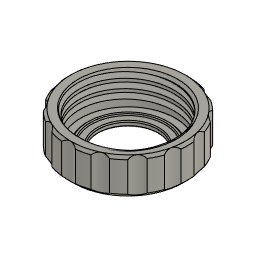
EnfamilTravelBottleNippleAdapter v7 (Autodesk Fusion 360 design; units mm, degrees)
Autodesk Fusion 360 part; units mm, degrees
sketch "Sketch1" plane through (0, 0, 0) normal (0, 1, 0) x (1, 0, 0)
  line L0 (0, 0) -> (0, -15) construction
  line L1 (12, 0) -> (12, -2)
  line L2 (14.7, -2) -> (14.7, -2.4)
  line L3 (14.7, -2.4) -> (16.3, -2.4)
  line L4 (16.3, -2.4) -> (16.3, -2)
  line L5 (16.3, -2) -> (19, -2)
  line L6 (19, -2) -> (19, -15)
  line L7 (19, -15) -> (24, -15)
  line L8 (24, -15) -> (24, 0)
  line L9 (24, 0) -> (12, 0)
  line L10 (12, -2) -> (14.7, -2)
  line L11 (0, -15) -> (0.379, -15)
  line L12 (0.379, -15) -> (19, -15) construction
  line L13 (0, 0) -> (12, 0) construction
  dimension "d1" = 15
  dimension "d2" = 12
  dimension "d3" = 19
  dimension "d4" = 1.6
  dimension "d5" = 0.4
  dimension "d6" = 2
  dimension "d7" = 5
  constraint coincident L0.start L13.start
  constraint vertical L0
  constraint parallel L0 L1
  constraint perpendicular L1 L3
  constraint perpendicular L3 L4
  constraint perpendicular L4 L5
  constraint perpendicular L3 L6
  constraint perpendicular L6 L7
  constraint perpendicular L7 L8
  constraint perpendicular L1 L9
  constraint perpendicular L2 L10
  constraint collinear L5 L10
  constraint equal L5 L10
  constraint perpendicular L0 L11
  constraint perpendicular L0 L12
  constraint perpendicular L1 L13
  measures "d1" distance of L0.start L0.end
  measures "d2" distance of L0 L1
  measures "d3" distance of L0 L6
  measures "d4" distance of L2.end L3.end
  measures "d5" distance of L2.start L2.end
  measures "d6" distance of L1.start L1.end
  measures "d7" distance of L6.end L7.end
revolve "Revolve1" add sketch "Sketch1" angle 360 about axis through (0, 0, 0) along (0, 0, 1)
ref_plane "WorkPlane1" through (0, 0, 4.5) normal (0, 0, 1) x (1, 0, 0)
chamfer "Chamfer1" distance 2 angle 45 1 edges at (-22.3759, -8.6788, 0)
chamfer "Chamfer1" distance 1 angle 45 1 edges at (-22.3759, -8.6788, 15)
chamfer "Chamfer1" distance 1 angle 45 1 edges at (-17.7142, -6.8707, 15)
chamfer "Chamfer1" distance 0.4 angle 45 2 edges at (-11.1879, -4.3394, 2) (-11.1879, -4.3394, 0)
chamfer "Chamfer1" distance 0.4 angle 45 2 edges at (-15.1969, -5.8943, 2.4) (-13.7052, -5.3157, 2.4)
sketch "Sketch5" plane through (0, 0, 15) normal (0, 0, 1) x (-1, 0, 0)
  circle A0 centre (0, 0) radius 23
  circle A1 centre (0, 0) radius 20
  circle A2 centre (0, 28) radius 5
  dimension "d22" = 10
  dimension "d23" = 28
  measures "d22" diameter of A2
  measures "d23" distance of A0.centre A2.centre
extrude "Extrude1" cut sketch "Sketch5" against normal through all contours A2
pattern_circular "C-Pattern1" count 14 over 360 about axis through (0, 0, 1.75) along (0, 0, 1) of "Extrude1"
coil "CoilPrimitive1" cut diameter 38 section triangle out size 2 outside turns 3.5 pitch 3.6 right hand placed x (1, 0, 0) y (0, 1, 0) z (0, 0, 1) at (0, 0, 4.5)
equation "d3 = ( 38 / 2 ) * 1 mm"
named bodies: "TravelBottleNippleAdapter"
